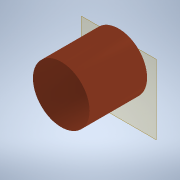
# Autodesk Inventor part: ManualKnob
Saved by Autodesk Inventor 2022 (Build 260153000, 153)
## iProperties
Created: 2023-05-09
Part Number: ManualKnob
Material: Generic
Document SubType Name: Modeling
Designer: UCadmin2
Density: 1 g/cm^3
Appearance: Copper - Polished
Author: UCadmin2
Autodesk Inventor part; units mm, degrees
ref_plane "YZ Plane" through (0, 0, 0) normal (1, 0, 0) x (0, 1, 0)
ref_plane "XZ Plane" through (0, 0, 0) normal (0, 1, 0) x (-1, 0, 0)
ref_plane "XY Plane" through (0, 0, 0) normal (0, 0, 1) x (1, 0, 0)
ref_plane "Work Plane1" through (0, 0, 0) normal (0, 0, 1) x (1, 0, 0)
sketch "Sketch1" plane through (0, 0, 0) normal (0, 0, 1) x (1, 0, 0)
  circle A0 centre (0, 6.35) radius 4 projected
  circle A1 centre (0, 6.35) radius 12.5
  point P0 (0, 0)
  dimension "d0" = 25
  constraints: 1 centre point, 1 coincident
  measures "d0" diameter of A1
extrude "Extrusion1" add sketch "Sketch1" along normal blind 25.4 contours A0 | A1
body "Solid1"
